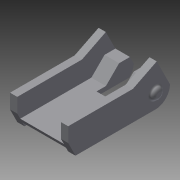
# Autodesk Inventor part: LegV2
Saved by Autodesk Inventor 2014 (Build 180170000, 170)
## iProperties
Created: 2014-04-23
Part Number: LegV2
Material: Generic
Document SubType Name: Modeling
Designer: Max
Density: 1 g/cm^3
Appearance: Default
Author: Max
Autodesk Inventor part; units mm, degrees
ref_plane "YZ Plane" through (0, 0, 0) normal (1, 0, 0) x (0, 1, 0)
ref_plane "XZ Plane" through (0, 0, 0) normal (0, 1, 0) x (-1, 0, 0)
ref_plane "XY Plane" through (0, 0, 0) normal (0, 0, 1) x (1, 0, 0)
sketch "Sketch2" plane through (0, 0, 0) normal (1, 0, 0) x (0, 1, 0)
  line L0 (0, 0) -> (12.7, 0) construction
  line L1 (12.7, 0) -> (12.7, 44.45) construction
  line L2 (12.7, 44.45) -> (0, 44.45) construction
  line L3 (0, 44.45) -> (0, 0) construction
  arc A0 (0, 6.35) -> (6.35, 0) centre (6.35, 6.35) ccw
  line L4 (6.35, 0) -> (6.35, 44.45) construction
  line L5 (6.35, 44.45) -> (0, 41.275)
  line L6 (0, 41.275) -> (0, 6.35)
  line L7 (6.35, 44.45) -> (6.35, 42.545)
  line L8 (6.35, 42.545) -> (1.905, 40.3225)
  line L9 (1.905, 40.3225) -> (1.905, 9.525)
  line L10 (6.35, 44.45) -> (12.7, 44.45)
  line L11 (6.35, 0) -> (12.7, 3.175)
  line L12 (12.7, 3.175) -> (12.7, 44.45)
  line L13 (6.35, 6.35) -> (6.35, 0)
  line L14 (6.35, 6.35) -> (1.905, 9.525)
  circle A1 centre (6.35, 6.35) radius 2.54
  line L15 (0, 16.1925) -> (12.7, 16.1925)
  line L16 (3.81, 0.5301) -> (3.81, 43.18)
  line L17 (1.905, 9.525) -> (1.905, 1.8152)
  line L18 (1.905, 40.3225) -> (1.905, 42.2275)
  line L19 (12.7, 16.1925) -> (17.907, 5.7785)
  line L20 (12.7, 3.175) -> (17.907, 5.7785)
  dimension "d2" = 12.7
  dimension "d3" = 44.45
  dimension "d4" = 12.7
  dimension "d5" = 3.175
  dimension "d6" = 1.905
  dimension "d7" = 1.905
  dimension "d8" = 3.175
  dimension "d9" = 3.175
  dimension "d10" = 5.08
  dimension "d11" = 16.1925
  dimension "d22" = 1.905
  constraints: 42 end point, 8 point on line, 7 perpendicular, 6 parallel, 4 point on circle, 3 tangent, 2 centre point, 2 collinear, 2 midpoint, 1 coincident, 1 horizontal
  measures "d2" distance of L2.end L1.end
  measures "d3" distance of L1.end L0.end
  measures "d4" diameter of A0
  measures "d5" vertical distance of L4.end L5.end
  measures "d6" distance of L4.end L7.end
  measures "d7" distance between parallel lines of L3 L9
  measures "d8" vertical distance of L4.start L11.end
  measures "d9" vertical distance of L13.start L9.end
  measures "d10" diameter of A1
  measures "d11" distance from line of L4.start L15
  measures "d22" distance between parallel lines of L9 L16
extrude "Extrusion1" add sketch "Sketch2" along normal mid plane 28.575 contours A1 L14 L13 | L13 L14 A1
extrude "Extrusion2" add sketch "Sketch2" along normal mid plane 25.4
extrude "Extrusion4" cut sketch "Sketch2" along normal mid plane 6.35 contours L6 L15 L9 L17 A0 | L17 L14 L16 A0 | L16 A1 L13 A0 | L9 L15 L16 L14 | L13 A1 L14 L16 L15 L12 L11 | L16 L14 A1 | A1 L14 L13 | L13 L14 A1
fillet "Fillet1" radius 1.5875 2 edges at (-14.2875, 3.81, 6.35) (14.2875, 3.81, 6.35)
fillet "Fillet2" radius 0.7937 4 edges at (-12.7, 3.81, 6.35) (-12.7001, 3.81, 6.35) (12.7001, 3.81, 6.35) (12.7, 3.81, 6.35)
sketch "Sketch3" plane through (0, 0, 0) normal (1, 0, 0) x (0, 1, 0)
  line L0 (12.7, 44.45) -> (12.7, 16.1925) projected
  line L1 (17.907, 5.7785) -> (6.35, 0) projected
  arc A0 (0, 6.35) -> (6.35, 0) centre (6.35, 6.35) ccw projected
  line L2 (0, 6.35) -> (0, 41.275) projected
  line L3 (0, 41.275) -> (6.35, 44.45) projected
  line L4 (6.35, 44.45) -> (12.7, 44.45) projected
  circle A1 centre (6.35, 6.35) radius 3.1976 projected
  circle A2 centre (6.35, 6.35) radius 3.1976 projected
  line L5 (3.81, 0.5301) -> (3.81, 43.18) projected
  line L6 (1.905, 40.3225) -> (1.905, 9.525) projected
  line L7 (1.905, 42.2275) -> (1.905, 1.8152)
  line L8 (0, 0) -> (1.905, 0)
  line L9 (1.905, 0) -> (1.905, 42.2275)
  line L10 (1.905, 42.2275) -> (0, 42.2275)
  line L11 (0, 42.2275) -> (0, 0)
  circle A3 centre (6.35, 6.35) radius 3.1976
  line L12 (9.5476, 44.45) -> (9.5476, 1.5988)
  line L13 (12.7, 44.45) -> (9.5476, 44.45)
  line L14 (9.5476, 44.45) -> (9.5476, 0)
  line L15 (9.5476, 0) -> (12.7, 0)
  line L16 (12.7, 0) -> (12.7, 44.45)
  line L17 (6.3337, 9.5475) -> (1.905, 9.525)
  circle A4 centre (6.35, 6.35) radius 3.1976
  line L18 (9.5476, 6.35) -> (9.5476, 0)
  line L19 (9.5476, 0) -> (1.905, 0)
  line L20 (9.5476, 7.1442) -> (9.5476, 44.45)
  line L21 (6.35, 44.45) -> (3.81, 43.18)
  line L22 (3.81, 12.0876) -> (3.81, 43.18)
  line L23 (1.905, 42.2275) -> (6.35, 44.45)
  line L24 (6.35, 44.45) -> (9.5476, 44.45)
  line L25 (9.5476, 44.45) -> (9.5476, 6.35)
  line L26 (9.5476, 6.35) -> (1.905, 13.9926)
  line L27 (12.7, 16.1925) -> (17.907, 5.7785) projected
  dimension "d25" = 1.905
  constraints: 40 end point, 8 collinear, 7 point on line, 6 tangent, 5 perpendicular, 5 vertical, 4 parallel, 3 point on circle, 2 coincident, 2 horizontal, 1 centre point, 7 other
  measures "d25" distance between parallel lines of L11 L9
extrude "Extrusion6" cut sketch "Sketch3" along normal mid plane 19.05 contours L0 L16 L1 L12 L4 | L27 L1 L16 | L12 A1 L26 L5 L3 L4 | L26 A1 | L7 L6 A0 L2 L3
equation "\"d7\" = d6"
equation "\"d22\" = d7"
body "Solid1"
